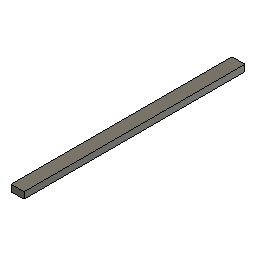
_BarBeam.5c540dc0-49b3-424c-a6fa-f8eb28995f75 (Autodesk Fusion 360 design; units mm, degrees)
Autodesk Fusion 360 part; units mm, degrees
sketch "Sketch1" plane through (0, 0, 0) normal (0, 0, 1) x (1, 0, 0)
  line L0 (6.481, 22.2416) -> (108.081, 22.2416)
  line L1 (108.081, 22.2416) -> (108.081, -28.5584)
  line L2 (108.081, -28.5584) -> (6.481, -28.5584)
  line L3 (6.481, -28.5584) -> (6.481, 22.2416)
  constraint horizontal L0
  constraint vertical L1
  constraint horizontal L2
  constraint vertical L3
extrude "Extrude1" add sketch "Sketch1" along normal blind 1731.45
